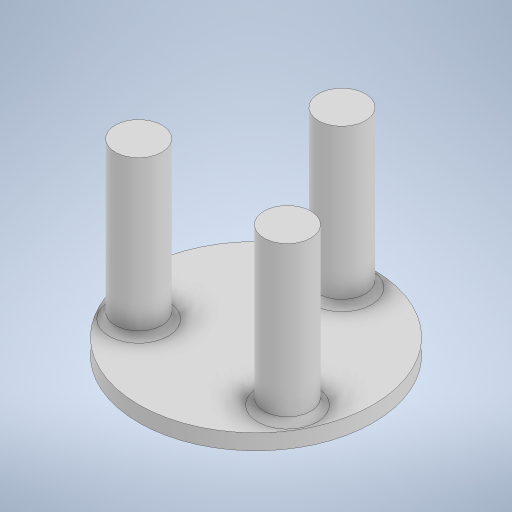
# Autodesk Inventor part: Part1
Saved by Autodesk Inventor 2023 (Build 270158000, 158)
## iProperties
Created: 2022-12-15
Part Number: Part1
Material: 一般
Document SubType Name: Modeling
Designer: yuta
Density: 1 g/cm^3
Appearance: 既定
Author: yuta
Autodesk Inventor part; units mm, degrees
ref_plane "YZ Plane" through (0, 0, 0) normal (1, 0, 0) x (0, 1, 0)
ref_plane "XZ Plane" through (0, 0, 0) normal (0, 1, 0) x (-1, 0, 0)
ref_plane "XY Plane" through (0, 0, 0) normal (0, 0, 1) x (1, 0, 0)
sketch "スケッチ1" plane through (0, 0, 0) normal (0, 1, 0) x (-1, 0, 0)
  circle A0 centre (0, 0) radius 75
  dimension "d0" = 150
  constraints: 1 centre point, 1 coincident
  measures "d0" diameter of A0
extrude "押し出し1" add sketch "スケッチ1" along normal blind 10
sketch "スケッチ2" plane through (0, 10, 0) normal (0, 1, 0) x (1, 0, 0)
  circle A0 centre (0, 55) radius 15
  circle A1 centre (-47.6314, -27.5) radius 15
  circle A2 centre (47.6314, -27.5) radius 15
  point P0 (0, 0)
  dimension "d3" = 30
  dimension "d4" = 55
  dimension "d7" = 360
  constraints: 3 centre point, 7 other
  measures "d3" diameter of A0
  measures "d4" distance of point (0, 0) A0.centre
extrude "押し出し2" add sketch "スケッチ2" along normal blind 100
fillet "フィレット1" radius 4 3 edges at (-62.6314, 10, 27.5) (32.6314, 10, 27.5) (-15, 10, -55)
